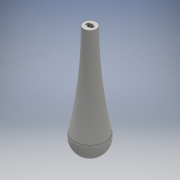
# Autodesk Inventor part: griff
Saved by Autodesk Inventor 2016 (Build 200138000, 138)
## iProperties
Created: 2016-06-02
Part Number: griff
Material: Generic
Document SubType Name: Modeling
Designer: Chris
Density: 1 g/cm^3
Appearance: Default
Author: Chris
Autodesk Inventor part; units mm, degrees
ref_plane "YZ Plane" through (0, 0, 0) normal (1, 0, 0) x (0, 1, 0)
ref_plane "XZ Plane" through (0, 0, 0) normal (0, 1, 0) x (-1, 0, 0)
ref_plane "XY Plane" through (0, 0, 0) normal (0, 0, 1) x (1, 0, 0)
sketch "Sketch2" plane through (0, 0, 0) normal (0, 1, 0) x (-1, 0, 0)
  line L0 (0, 0) -> (0, -70)
  arc A0 (-9.802, -58.0198) -> (0, -70) centre (0, -60) ccw
  line L1 (0, 0) -> (-4, 0)
  arc A1 (-9.802, -58.0198) -> (-4, 0) centre (-297, 0) ccw
  point P0 (0, -70)
  dimension "d1" = 70
  dimension "d2" = 4
  dimension "d10" = 10
  constraints: 5 point on circle, 4 end point, 3 coincident, 2 centre point, 2 point on line, 1 horizontal, 1 horizontal alignment, 1 tangent, 1 vertical
  measures "d1" distance of L0.start L0.end
  measures "d2" distance of L0.start L1.end
  measures "d10" distance edge to line of A0 L0
revolve "Revolution1" add sketch "Sketch2" angle 360 about axis through (0, 0, 0) along (0, 0, -1)
sketch "Sketch3" plane through (0, 0, 0) normal (0, 0, 1) x (1, 0, 0)
  circle A0 centre (0, 0) radius 1.4
  line L0 (2, 0.85) -> (-2, 0.85)
  line L1 (-2, 0.85) -> (-2, -0.85)
  line L2 (-2, -0.85) -> (2, -0.85)
  line L3 (2, -0.85) -> (2, 0.85)
  line L4 (2, 0.85) -> (-2, -0.85) construction
  line L5 (-2, 0.85) -> (2, -0.85) construction
  dimension "d5" = 2.8
  dimension "d6" = 4
  dimension "d7" = 1.7
  constraints: 12 end point, 2 midpoint, 2 parallel, 1 centre point, 1 coincident, 1 horizontal, 1 perpendicular
  measures "d5" diameter of A0
  measures "d6" distance of L2.end L1.end
  measures "d7" distance of L1.end L0.end
extrude "Extrusion1" cut sketch "Sketch3" against normal blind 30
body "Solid1"
